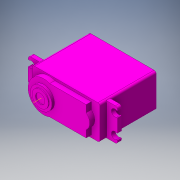
# Autodesk Inventor part: servo
Saved by Autodesk Inventor 2016 (Build 200138000, 138)
## iProperties
Created: 2016-02-10
Part Number: servo
Material: Generic
Document SubType Name: Modeling
Designer: RoksBot
Density: 1 g/cm^3
Appearance: Magenta
Author: RoksBot
Autodesk Inventor part; units mm, degrees
ref_plane "YZ Plane" through (0, 0, 0) normal (1, 0, 0) x (0, 1, 0)
ref_plane "XZ Plane" through (0, 0, 0) normal (0, 1, 0) x (-1, 0, 0)
sketch "Sketch1" plane through (0, 0, 0) normal (0, 0, 1) x (1, 0, 0)
  line L0 (-19.9263, -9.8806) -> (19.9263, -9.8806)
  line L1 (19.9263, -9.8806) -> (19.9263, 9.8806)
  line L2 (19.9263, 9.8806) -> (-19.9263, 9.8806)
  line L3 (-19.9263, 9.8806) -> (-19.9263, -9.8806)
  line L4 (-19.9263, -9.8806) -> (19.9263, 9.8806) construction
  line L5 (19.9263, -9.8806) -> (-19.9263, 9.8806) construction
  point P0 (0, 0)
  dimension "d0" = 39.8526
  dimension "d1" = 19.7612
  constraints: 12 end point, 2 midpoint, 2 parallel, 1 horizontal, 1 perpendicular
  measures "d0" distance of L1.end L2.end
  measures "d1" distance of L2.end L0.start
extrude "Extrusion1" add sketch "Sketch1" along normal blind 33.1724
ref_plane "Work Plane1" through (0, 0, 29.21) normal (0, 0, 1) x (1, 0, 0)
sketch "Sketch2" plane through (0, 0, 29.21) normal (0, 0, 1) x (1, 0, 0)
  line L0 (-19.9263, -9.8806) -> (19.9263, -9.8806) projected
  line L1 (-19.9263, 9.8806) -> (-19.9263, -9.8806) projected
  line L2 (19.9263, 9.8806) -> (-19.9263, 9.8806) projected
  line L3 (19.9263, -9.8806) -> (19.9263, 9.8806) projected
  line L4 (26.2763, -9.4869) -> (-26.2763, -9.4869)
  line L5 (-26.2763, -9.4869) -> (-26.2763, 9.4869)
  line L6 (-26.2763, 9.4869) -> (26.2763, 9.4869)
  line L7 (26.2763, 9.4869) -> (26.2763, -9.4869)
  line L8 (26.2763, -9.4869) -> (-26.2763, 9.4869) construction
  line L9 (-26.2763, -9.4869) -> (26.2763, 9.4869) construction
  point P0 (0, 0)
  dimension "d5" = 52.5526
  dimension "d6" = 18.9738
  constraints: 12 end point, 2 midpoint, 2 parallel, 1 horizontal, 1 perpendicular
  measures "d5" distance of L5.end L6.end
  measures "d6" distance of L4.end L5.end
extrude "Extrusion2" add sketch "Sketch2" against normal blind 2.3114 contours L4 L5 L6 L1 | L1 L6 L3 L4 | L3 L6 L7 L4
fillet "Fillet1" radius 1.27 8 edges at (19.9263, 9.8806, 16.5862) (-19.9263, 9.8806, 16.5862) (19.9263, -9.8806, 16.5862) (-19.9263, -9.8806, 16.5862) (26.2763, 9.4869, 28.0543) (26.2763, -9.4869, 28.0543) (-26.2763, 9.4869, 28.0543) (-26.2763, -9.4869, 28.0543)
sketch "Sketch3" plane through (0, 0, 29.21) normal (0, 0, 1) x (1, 0, 0)
  circle A0 centre (-24.6761, 5.7404) radius 2.0193
  circle A1 centre (-24.6761, -5.7404) radius 2.0193
  circle A2 centre (24.6761, 5.7404) radius 2.0193
  circle A3 centre (24.6761, -5.7404) radius 2.0193
  line L0 (-25.0063, 9.4869) -> (-19.5755, 9.4869) projected
  line L1 (-19.5755, -9.4869) -> (-25.0063, -9.4869) projected
  line L2 (-26.2763, -8.2169) -> (-26.2763, 8.2169) projected
  line L3 (26.2763, 8.2169) -> (26.2763, -8.2169) projected
  point P0 (0, 0)
  dimension "d10" = 4.0386
  dimension "d11" = 1.7272
  dimension "d12" = 1.7272
  dimension "d13" = 45.3136
  dimension "d14" = 1.6002
  dimension "d15" = 1.6002
  constraints: 4 centre point, 3 equal radius, 2 horizontal alignment, 2 vertical alignment
  measures "d10" diameter of A2
  measures "d11" distance edge to line of A0 L0
  measures "d12" distance edge to line of A1 L1
  measures "d14" distance from line of L2 A0.centre
  measures "d15" distance from line of L3 A2.centre
extrude "Extrusion3" cut sketch "Sketch3" against normal blind 2.3114
fillet "Fillet2" radius 0.3175 8 edges at (26.2763, 6.972, 28.0543) (26.2763, 4.5088, 28.0543) (26.2763, -4.5088, 28.0543) (26.2763, -6.972, 28.0543) (-26.2763, -4.5088, 28.0543) (-26.2763, -6.972, 28.0543) (-26.2763, 6.972, 28.0543) (-26.2763, 4.5088, 28.0543)
sketch "Sketch4" plane through (0, 0, 33.1724) normal (0, 0, 1) x (1, 0, 0)
  circle A0 centre (-10.1981, 0) radius 9.2202
  line L0 (-11.2128, -8.509) -> (14.8463, -8.509)
  line L1 (14.8463, -8.509) -> (14.8463, 8.509)
  line L2 (14.8463, 8.509) -> (-11.2128, 8.509)
  line L3 (-11.2128, 8.509) -> (-11.2128, -8.509)
  line L4 (-11.2128, -8.509) -> (14.8463, 8.509) construction
  line L5 (14.8463, -8.509) -> (-11.2128, 8.509) construction
  arc A1 (14.8463, -4.318) -> (14.8463, 4.318) centre (11.2744, 0) ccw
  arc A2 (-19.9263, -8.6106) -> (-18.6563, -9.8806) centre (-18.6563, -8.6106) ccw projected
  line L6 (-18.6563, -9.8806) -> (18.6563, -9.8806) projected
  arc A3 (18.6563, -9.8806) -> (19.9263, -8.6106) centre (18.6563, -8.6106) ccw projected
  line L7 (19.9263, -8.6106) -> (19.9263, 8.6106) projected
  arc A4 (19.9263, 8.6106) -> (18.6563, 9.8806) centre (18.6563, 8.6106) ccw projected
  line L8 (18.6563, 9.8806) -> (-18.6563, 9.8806) projected
  arc A5 (-18.6563, 9.8806) -> (-19.9263, 8.6106) centre (-18.6563, 8.6106) ccw projected
  line L9 (-19.9263, 8.6106) -> (-19.9263, -8.6106) projected
  point P0 (0, 0)
  point P1 (1.8167, 0)
  point P2 (1.8167, 0)
  point P3 (1.8167, 0)
  dimension "d19" = 18.4404
  dimension "d20" = 0.508
  dimension "d21" = 17.018
  dimension "d22" = 5.08
  dimension "d23" = 8.636
  dimension "d24" = 2.032
  constraints: 12 end point, 4 midpoint, 3 horizontal alignment, 2 centre point, 2 parallel, 2 point on circle, 2 point on line, 1 horizontal, 1 perpendicular
  measures "d19" diameter of A0
  measures "d20" distance edge to line of A0 L9
  measures "d21" distance between parallel lines of L0 L2
  measures "d22" distance between parallel lines of L1 L7
  measures "d23" distance of A1.start A1.end
  measures "d24" distance edge to line of A1 L1
extrude "Extrusion4" add sketch "Sketch4" along normal blind 3.048 contours A0 L0 L3 L2 | A0 L2 L1 L0 | L2 L3 L0 A0 | A1 L1
sketch "Sketch5" plane through (0, 0, 36.2204) normal (0, 0, 1) x (1, 0, 0)
  line L0 (-6.6472, -8.509) -> (14.8463, -8.509) projected
  line L1 (14.8463, -8.509) -> (14.8463, -4.318) projected
  arc A0 (14.8463, -4.318) -> (14.8463, 4.318) centre (11.2744, 0) ccw projected
  line L2 (14.8463, 4.318) -> (14.8463, 8.509) projected
  line L3 (14.8463, 8.509) -> (-6.6472, 8.509) projected
  arc A1 (-6.6472, 8.509) -> (-6.6472, -8.509) centre (-10.1981, 0) ccw projected
  circle A2 centre (-10.1981, 0) radius 6.35
  point P0 (0, 0)
  dimension "d27" = 12.7
  constraints: 1 centre point, 1 coincident
  measures "d27" diameter of A2
extrude "Extrusion5" add sketch "Sketch5" along normal blind 1.524 contours A2
sketch "Sketch6" plane through (-10.1981, 0, 37.7444) normal (0, 0, 1) x (1, 0, 0)
  circle A0 centre (0, 0) radius 6.35 projected
  circle A1 centre (0, 0) radius 4.826
  circle A2 centre (0, 0) radius 2.794
  point P0 (10.1981, 0)
  dimension "d30" = 9.652
  dimension "d31" = 5.588
  constraints: 2 centre point, 2 coincident
  measures "d30" diameter of A1
  measures "d31" diameter of A2
extrude "Extrusion6" add sketch "Sketch6" along normal blind 0.508 contours A1
sketch "Sketch7" plane through (-19.9263, -8.6106, 0) normal (-1, 0, 0) x (0, 0, 1)
  line L0 (0.762, 11.7856) -> (4.572, 11.7856)
  line L1 (4.572, 11.7856) -> (4.572, 5.4356)
  line L2 (4.572, 5.4356) -> (0.762, 5.4356)
  line L3 (0.762, 5.4356) -> (0.762, 11.7856)
  line L4 (0.762, 11.7856) -> (4.572, 5.4356) construction
  line L5 (4.572, 11.7856) -> (0.762, 5.4356) construction
  line L6 (26.8986, 0) -> (0, 0) projected
  line L7 (26.8986, 0) -> (26.8986, 17.2212) projected
  line L8 (0, 17.2212) -> (26.8986, 17.2212) projected
  line L9 (0, 17.2212) -> (0, 0) projected
  point P0 (0, 8.6106)
  point P1 (2.667, 8.6106)
  point P2 (2.667, 8.6106)
  point P3 (0, 8.6106)
  dimension "d34" = 6.35
  dimension "d35" = 3.81
  dimension "d36" = 0.762
  constraints: 12 end point, 4 midpoint, 2 parallel, 1 horizontal, 1 horizontal alignment, 1 perpendicular
  measures "d34" distance of L0.end L1.end
  measures "d35" distance of L1.end L2.end
  measures "d36" distance between parallel lines of L9 L3
extrude "Extrusion7" add sketch "Sketch7" along normal blind 1.27 draft -10 contours L0 L1 L2 L3
sketch "Sketch8" plane through (-21.1963, -8.6106, 0) normal (-1, 0, 0) x (0, 0, 1)
  circle A0 centre (2.667, 8.6106) radius 0.635
  circle A1 centre (2.667, 9.8806) radius 0.635
  circle A2 centre (2.667, 7.3406) radius 0.635
  line L0 (4.3481, 11.5617) -> (4.3481, 5.6595) projected
  line L1 (0.9859, 11.5617) -> (4.3481, 11.5617) projected
  line L2 (0.9859, 5.6595) -> (0.9859, 11.5617) projected
  line L3 (4.3481, 5.6595) -> (0.9859, 5.6595) projected
  point P0 (0, 8.6106)
  point P1 (2.667, 11.5617)
  dimension "d39" = 1.27
  constraints: 4 equal radius, 3 centre point, 3 vertical alignment, 1 horizontal alignment, 1 midpoint
  measures "d39" diameter of A1
extrude "Extrusion8" add sketch "Sketch8" along normal blind 1.27 contours A0 | A2 | A1
equation "\"d12\" = d11"
equation "\"d14\" = d15"
body "Solid1"
